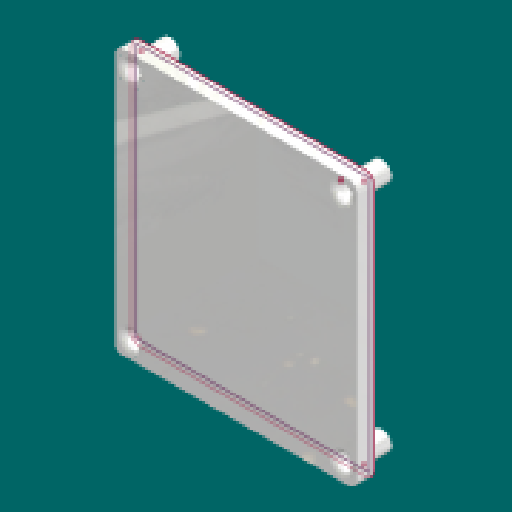
# Autodesk Inventor part: Part_uno_bawah
Saved by Autodesk Inventor 2025.2 (Build 292293000, 293)
## iProperties
Created: 2025-05-06
Part Number: Part_uno_bawah
Material: PPS Plastic
Document SubType Name: Modeling
Designer: ia088
Density: 1.637 g/cm^3
Appearance: Smooth - White
Author: ia088
Autodesk Inventor part; units mm, degrees
ref_plane "YZ Plane" through (0, 0, 0) normal (1, 0, 0) x (0, 1, 0)
ref_plane "XZ Plane" through (0, 0, 0) normal (0, 1, 0) x (-1, 0, 0)
ref_plane "XY Plane" through (0, 0, 0) normal (0, 0, 1) x (1, 0, 0)
ref_plane "Work Plane1" through (0, 0, 0) normal (0, 0, 1) x (1, 0, 0)
sketch "Sketch1" plane through (0, 0, 0) normal (0, 0, 1) x (1, 0, 0)
  line L0 (0, 0) -> (0, -66.04) projected
  line L1 (-53.34, 0) -> (0, 0) projected
  line L2 (-53.34, -66.04) -> (-53.34, 0) projected
  line L3 (-40.386, -66.04) -> (-53.34, -66.04) projected
  line L4 (-37.846, -68.58) -> (-40.386, -66.04) projected
  line L5 (-5.08, -68.58) -> (-37.846, -68.58) projected
  line L6 (-2.54, -66.04) -> (-5.08, -68.58) projected
  line L7 (0, -66.04) -> (-2.54, -66.04) projected
  circle A0 centre (-2.54, -33.02) radius 0.4 projected
  circle A1 centre (-2.54, -35.56) radius 0.4 projected
  circle A2 centre (-2.54, -38.1) radius 0.4 projected
  circle A3 centre (-2.54, -40.64) radius 0.4 projected
  circle A4 centre (-2.54, -43.18) radius 0.4 projected
  circle A5 centre (-2.54, -45.72) radius 0.4 projected
  circle A6 centre (-2.54, -50.8) radius 0.4 projected
  circle A7 centre (-2.54, -53.34) radius 0.4 projected
  circle A8 centre (-2.54, -55.88) radius 0.4 projected
  circle A9 centre (-2.54, -58.42) radius 0.4 projected
  circle A10 centre (-2.54, -60.96) radius 0.4 projected
  circle A11 centre (-2.54, -63.5) radius 0.4 projected
  circle A12 centre (-50.8, -23.876) radius 0.4 projected
  circle A13 centre (-50.8, -26.416) radius 0.4 projected
  circle A14 centre (-50.8, -28.956) radius 0.4 projected
  circle A15 centre (-50.8, -31.496) radius 0.4 projected
  circle A16 centre (-50.8, -34.036) radius 0.4 projected
  circle A17 centre (-50.8, -36.576) radius 0.4 projected
  circle A18 centre (-50.8, -39.116) radius 0.4 projected
  circle A19 centre (-50.8, -41.656) radius 0.4 projected
  circle A20 centre (-50.8, -50.8) radius 0.4 projected
  circle A21 centre (-50.8, -53.34) radius 0.4 projected
  circle A22 centre (-50.8, -55.88) radius 0.4 projected
  circle A23 centre (-50.8, -58.42) radius 0.4 projected
  circle A24 centre (-50.8, -60.96) radius 0.4 projected
  circle A25 centre (-50.8, -63.5) radius 0.4 projected
  circle A26 centre (-12.573, -62.865) radius 0.4 projected
  circle A27 centre (-20.193, -62.865) radius 0.4 projected
  circle A28 centre (-12.573, -60.325) radius 0.4 projected
  circle A29 centre (-20.193, -60.325) radius 0.4 projected
  circle A30 centre (-12.573, -57.785) radius 0.4 projected
  circle A31 centre (-20.193, -57.785) radius 0.4 projected
  circle A32 centre (-12.573, -55.245) radius 0.4 projected
  circle A33 centre (-20.193, -55.245) radius 0.4 projected
  circle A34 centre (-12.573, -52.705) radius 0.4 projected
  circle A35 centre (-20.193, -52.705) radius 0.4 projected
  circle A36 centre (-12.573, -50.165) radius 0.4 projected
  circle A37 centre (-20.193, -50.165) radius 0.4 projected
  circle A38 centre (-12.573, -47.625) radius 0.4 projected
  circle A39 centre (-20.193, -47.625) radius 0.4 projected
  circle A40 centre (-12.573, -45.085) radius 0.4 projected
  circle A41 centre (-20.193, -45.085) radius 0.4 projected
  circle A42 centre (-12.573, -42.545) radius 0.4 projected
  circle A43 centre (-20.193, -42.545) radius 0.4 projected
  circle A44 centre (-12.573, -40.005) radius 0.4 projected
  circle A45 centre (-20.193, -40.005) radius 0.4 projected
  circle A46 centre (-12.573, -37.465) radius 0.4 projected
  circle A47 centre (-20.193, -37.465) radius 0.4 projected
  circle A48 centre (-12.573, -34.925) radius 0.4 projected
  circle A49 centre (-20.193, -34.925) radius 0.4 projected
  circle A50 centre (-12.573, -32.385) radius 0.4 projected
  circle A51 centre (-20.193, -32.385) radius 0.4 projected
  circle A52 centre (-12.573, -29.845) radius 0.4 projected
  circle A53 centre (-20.193, -29.845) radius 0.4 projected
  circle A54 centre (-26.162, -16.383) radius 0.5 projected
  circle A55 centre (-26.162, -21.463) radius 0.5 projected
  circle A56 centre (-39.878, -18.288) radius 0.4 projected
  circle A57 centre (-39.878, -20.828) radius 0.4 projected
  circle A58 centre (-42.418, -20.828) radius 0.4 projected
  circle A59 centre (-42.418, -18.288) radius 0.4 projected
  circle A60 centre (-44.958, -15.748) radius 0.4 projected
  circle A61 centre (-44.958, -18.288) radius 0.4 projected
  circle A62 centre (-44.958, -20.828) radius 0.4 projected
  circle A63 centre (-47.498, -20.828) radius 0.4 projected
  circle A64 centre (-47.498, -18.288) radius 0.4 projected
  circle A65 centre (-47.498, -15.748) radius 0.4 projected
  circle A66 centre (-30.43, -63.64) radius 0.4 projected
  circle A67 centre (-27.89, -63.64) radius 0.4 projected
  circle A68 centre (-25.35, -63.64) radius 0.4 projected
  circle A69 centre (-25.35, -66.18) radius 0.4 projected
  circle A70 centre (-27.89, -66.18) radius 0.4 projected
  circle A71 centre (-30.43, -66.18) radius 0.4 projected
  circle A72 centre (-50.8, -48.26) radius 0.4 projected
  circle A73 centre (-50.8, -21.336) radius 0.4 projected
  circle A74 centre (-50.8, -45.72) radius 0.4 projected
  circle A75 centre (-2.54, -30.48) radius 0.4 projected
  circle A76 centre (-50.8, -18.796) radius 0.4 projected
  circle A77 centre (-2.54, -27.94) radius 0.4 projected
  circle A78 centre (-50.8, -15.24) radius 1.5875 projected
  circle A79 centre (-2.54, -13.97) radius 1.5875 projected
  circle A80 centre (-35.56, -66.04) radius 1.5875 projected
  circle A81 centre (-7.62, -66.04) radius 1.5875 projected
  line L8 (-43.58, 6.35) -> (-32.46, 6.35) projected
  line L9 (-44.04, 6.35) -> (-43.58, 6.35) projected
  line L10 (-32, 6.35) -> (-32.46, 6.35) projected
  line L11 (-32, 5.94) -> (-32, 6.35) projected
  line L12 (-32, 3.85) -> (-32, 5.94) projected
  line L13 (-32, 3.75) -> (-32, -2.65) projected
  line L14 (-32, 5.89) -> (-32, 3.75) projected
  line L15 (-44.04, -2.65) -> (-44.04, 3.75) projected
  line L16 (-44.04, 3.75) -> (-44.04, 5.89) projected
  line L17 (-44.04, 6.35) -> (-44.04, 5.94) projected
  line L18 (-44.04, 5.94) -> (-44.04, 3.85) projected
  line L19 (-53.34, 6.35) -> (-58.34, 6.35)
  line L20 (-58.34, 6.35) -> (31.66, 6.35)
  line L21 (31.66, 6.35) -> (31.66, -73.65)
  line L22 (31.66, -73.65) -> (-58.34, -73.65)
  line L23 (-58.34, -73.65) -> (-58.34, 6.35)
  dimension "d0" = 5
  dimension "d2" = 90
  dimension "d3" = 80
  constraints: 10 end point, 2 horizontal, 2 parallel, 1 perpendicular
  measures "d0" distance of L19.start L19.end
  measures "d2" distance of L21.end L22.end
  measures "d3" distance of L20.end L21.end
ref_plane "Work Plane2" through (0, 0, 0) normal (0, 0, 1) x (1, 0, 0)
sketch "Sketch2" plane through (0, 0, 0) normal (0, 0, 1) x (1, 0, 0)
  point P0 (0, 0)
extrude "Extrusion1" add sketch "Sketch1" along normal blind 5 contours L1 L13 L14 L12 L11 L20 L21 L22 L23 L19 L17 L18 L16 L15 L2 L3 L4 L5 L6 L7 L0 | L0 L7 L6 L5 L4 L3 L2 L1 | L1 L15 L16 L18 L17 L9 L8 L10 L11 L12 L14 L13 | A0 | A1 | A2 | A3 | A4 | A5 | A6 | A7 | A8 | A9 | A10 | A11 | A12 | A13 | A14 | A15 | A16 | A17 | A18 | A19 | A20 | A21 | A22 | A23 | A24 | A25 | A26 | A27 | A28 | A29 | A30 | A31 | A32 | A33 | A34 | A35 | A36 | A37 | A38 | A39 | A40 | A41 | A42 | A43 | A44 | A45 | A46 | A47 | A48 | A49 | A50 | A51 | A52 | A53 | A54 | A55 | A56 | A57 | A58 | A59 | A60 | A61 | A62 | A63 | A64 | A65 | A66 | A67 | A68 | A69 | A70 | A71 | A72 | A73 | A74 | A75 | A76 | A77 | A78 | A79 | A80 | A81
sketch "Sketch3" plane through (0, 0, 0) normal (0, 0, -1) x (-1, 0, 0)
  circle A0 centre (2.54, -13.97) radius 1.5875 projected
  circle A1 centre (50.8, -15.24) radius 1.5875 projected
  circle A2 centre (35.56, -66.04) radius 1.5875 projected
  circle A3 centre (7.62, -66.04) radius 1.5875 projected
  line L0 (53.34, 0) -> (0, 0) construction
  line L1 (0, 0) -> (0, -66.04) construction
  line L2 (0, -66.04) -> (2.54, -66.04) construction
  line L3 (2.54, -66.04) -> (5.08, -68.58) construction
  line L4 (5.08, -68.58) -> (37.846, -68.58) construction
  line L5 (37.846, -68.58) -> (40.386, -66.04) construction
  line L6 (40.386, -66.04) -> (53.34, -66.04) construction
  line L7 (53.34, -66.04) -> (53.34, 0) construction
  line L8 (-0.3, 0.3) -> (53.64, 0.3)
  line L9 (53.64, 0.3) -> (53.64, -66.34)
  line L10 (53.64, -66.34) -> (40.5103, -66.34)
  line L11 (40.5103, -66.34) -> (37.9703, -68.88)
  line L12 (37.9703, -68.88) -> (4.9557, -68.88)
  line L13 (4.9557, -68.88) -> (2.4157, -66.34)
  line L14 (2.4157, -66.34) -> (-0.3, -66.34)
  line L15 (-0.3, -66.34) -> (-0.3, 0.3)
  circle A4 centre (2.54, -13.97) radius 1.2875
  circle A5 centre (50.8, -15.24) radius 1.2875
  circle A6 centre (7.62, -66.04) radius 1.2875
  circle A7 centre (35.56, -66.04) radius 1.2875
  dimension "d6" = 0.3
  dimension "d9" = 0.3
  dimension "d10" = 0.3
  dimension "d11" = 0.3
  dimension "d12" = 0.3
  constraints: 16 end point, 4 centre point, 7 other
  measures "d6" distance between parallel lines of L0 L8
  measures "d9" radial gap between concentric circles of A0 A4
  measures "d10" radial gap between concentric circles of A1 A5
  measures "d11" radial gap between concentric circles of A3 A6
  measures "d12" radial gap between concentric circles of A2 A7
extrude "Extrusion2" cut sketch "Sketch3" against normal blind 3 contours A0 | A1 | A2 | A3 | L8 L9 L10 L11 L12 L13 L14 L15
sketch "Sketch4" plane through (0, 0, 0) normal (0, 0, -1) x (-1, 0, 0)
  circle A0 centre (7.62, -66.04) radius 1.2875 projected
  circle A1 centre (2.54, -13.97) radius 1.2875 projected
  circle A2 centre (50.8, -15.24) radius 1.2875 projected
  circle A3 centre (35.56, -66.04) radius 1.2875 projected
  point P0 (0, 0)
extrude "Extrusion3" add sketch "Sketch4" along normal blind 3
fillet "Fillet1" radius 1 4 edges at (-6.3325, -66.04, 3) (-34.2725, -66.04, 3) (-1.2525, -13.97, 3) (-49.5125, -15.24, 3)
sketch "Sketch5" plane through (0, 0, 0) normal (0, 0, -1) x (-1, 0, 0)
  line L0 (4.9557, -68.88) -> (2.4157, -66.34) projected
  line L1 (2.4157, -66.34) -> (-0.3, -66.34) projected
  line L2 (-0.3, -66.34) -> (-0.3, 0.3) projected
  line L3 (-0.3, 0.3) -> (53.64, 0.3) projected
  line L4 (53.64, 0.3) -> (53.64, -66.34) projected
  line L5 (53.64, -66.34) -> (40.5103, -66.34) projected
  line L6 (40.5103, -66.34) -> (37.9703, -68.88) projected
  line L7 (37.9703, -68.88) -> (4.9557, -68.88) projected
  line L8 (-31.66, 6.35) -> (58.34, 6.35) projected
  line L9 (-31.66, -73.65) -> (-31.66, 6.35) projected
  line L10 (58.34, -73.65) -> (-31.66, -73.65) projected
  line L11 (58.34, 6.35) -> (58.34, -73.65) projected
  line L12 (56.84, 4.85) -> (-30.16, 4.85)
  line L13 (-30.16, 4.85) -> (-30.16, -72.15)
  line L14 (-30.16, -72.15) -> (56.84, -72.15)
  line L15 (56.84, -72.15) -> (56.84, 4.85)
  line L16 (55.14, 1.8) -> (-1.8, 1.8)
  line L17 (-1.8, 1.8) -> (-1.8, -67.84)
  line L18 (-1.8, -67.84) -> (1.7944, -67.84)
  line L19 (1.7944, -67.84) -> (4.3344, -70.38)
  line L20 (4.3344, -70.38) -> (38.5916, -70.38)
  line L21 (38.5916, -70.38) -> (41.1316, -67.84)
  line L22 (41.1316, -67.84) -> (55.14, -67.84)
  line L23 (55.14, -67.84) -> (55.14, 1.8)
  point P0 (0, 0)
  dimension "d16" = 1.5
  dimension "d17" = 1.5
  constraints: 24 end point, 10 other
  measures "d16" distance between parallel lines of L8 L12
  measures "d17" distance between parallel lines of L3 L16
extrude "Extrusion4" cut sketch "Sketch5" against normal blind 3 contours L15 L14 L13 L12
sketch "Sketch6" plane through (-58.34, -73.65, 0) normal (-1, 0, 0) x (0, 0, 1)
  line L0 (0, 80) -> (0, 0) projected
  line L1 (0, 0) -> (5, 0) projected
  line L2 (5, 80) -> (5, 0) projected
  line L3 (0, 80) -> (5, 80) projected
  point P0 (0, 73.65)
extrude "Extrusion5" add sketch "Sketch6" along normal blind 5
sketch "Sketch7" plane through (0, 0, 0) normal (0, 0, -1) x (-1, 0, 0)
  line L0 (63.34, 6.35) -> (63.34, -73.65) projected
  line L1 (56.84, 4.85) -> (56.84, -72.15) projected
  line L2 (56.84, -72.15) -> (61.84, -72.15)
  line L3 (61.84, -72.15) -> (61.84, 4.85)
  line L4 (61.84, 4.85) -> (56.84, 4.85)
  point P0 (0, 0)
  dimension "d23" = 5
  constraints: 6 end point, 2 perpendicular, 1 parallel
  measures "d23" distance of L1.end L2.end
extrude "Extrusion6" cut sketch "Sketch7" against normal up to surface (3 mm away)
sketch "Sketch8" plane through (0, 0, 3) normal (0, 0, -1) x (-1, 0, 0)
  line L0 (-30.16, -72.15) -> (-30.16, 4.85) projected
  line L1 (61.84, -72.15) -> (-30.16, -72.15) projected
  line L2 (61.84, 4.85) -> (-30.16, 4.85) projected
  line L3 (55.14, -67.84) -> (55.14, 1.8) projected
  line L4 (61.84, -72.15) -> (55.84, -72.15)
  line L5 (61.84, -66.15) -> (61.84, -72.15)
  line L6 (61.84, -72.15) -> (55.14, -72.15)
  line L7 (55.14, -72.15) -> (55.14, -65.45)
  line L8 (55.14, -65.45) -> (61.84, -65.45)
  line L9 (61.84, -65.45) -> (61.84, -72.15)
  circle A0 centre (58.49, -68.8) radius 3
  circle A1 centre (58.49, -68.8) radius 1.6
  line L10 (61.84, -72.15) -> (15.84, -72.15)
  line L11 (15.84, -72.15) -> (15.84, 4.85)
  line L12 (-30.16, -72.15) -> (61.84, -72.15)
  circle A2 centre (-26.81, -68.8) radius 3
  line L13 (15.84, -33.65) -> (-30.16, -33.65)
  circle A3 centre (58.49, 1.5) radius 3
  circle A4 centre (58.49, 1.5) radius 1.6
  circle A5 centre (-26.81, 1.5) radius 3
  circle A6 centre (-26.81, -68.8) radius 1.6
  circle A7 centre (-26.81, 1.5) radius 1.6
  point P0 (0, 0)
  dimension "d30" = 6.7
  dimension "d31" = 6
  dimension "d32" = 3.2
  dimension "d33" = 46
  dimension "d34" = 3.2
  dimension "d35" = 3.2
  constraints: 20 end point, 8 centre point, 6 symmetric about line, 4 coincident, 4 midpoint, 2 horizontal, 2 parallel, 1 perpendicular, 1 point on line, 4 other
  measures "d30" distance of L6.end L7.end
  measures "d31" diameter of A0
  measures "d32" diameter of A1
  measures "d33" distance of L1.start L10.end
  measures "d34" diameter of A6
  measures "d35" diameter of A7
extrude "Extrusion7" add sketch "Sketch8" along normal blind 10 contours A0 | A1 | A2 | A3 | A4 | A5 | A6 | A7
sketch "Sketch9" plane through (-58.49, -68.8, -7) normal (0, 0, -1) x (-1, 0, 0)
  circle A0 centre (0, 0) radius 3 projected
  circle A1 centre (0, 0) radius 2
  circle A2 centre (0, 70.3) radius 3 projected
  circle A3 centre (-85.3, 70.3) radius 3 projected
  circle A4 centre (-85.3, 0) radius 3 projected
  circle A5 centre (0, 70.3) radius 2
  circle A6 centre (-85.3, 70.3) radius 2
  circle A7 centre (-85.3, 0) radius 2
  point P0 (-58.49, 68.8)
  dimension "d38" = 1
  dimension "d39" = 1
  dimension "d40" = 1
  dimension "d41" = 1
  constraints: 4 centre point
  measures "d38" radial gap between concentric circles of A0 A1
  measures "d39" radial gap between concentric circles of A2 A5
  measures "d40" radial gap between concentric circles of A3 A6
  measures "d41" radial gap between concentric circles of A4 A7
extrude "Extrusion8" cut sketch "Sketch9" against normal up to surface (12 mm away) contours A1 | A5 | A6 | A7
fillet "Fillet3" radius 2 4 edges at (-56.49, 1.5, 5) (-56.49, -68.8, 5) (28.81, -68.8, 5) (28.81, 1.5, 5)
fillet "Fillet4" radius 1 3 edges at (-55.49, 1.5, 3) (29.81, 1.5, 3) (29.81, -68.8, 3)
sketch "Sketch10" plane through (26.81, -68.8, -7) normal (0, 0, -1) x (-1, 0, 0)
  line L0 (25.01, 70.6) -> (25.01, 0.96) projected
  line L1 (25.01, 0.96) -> (16.81, 0.96)
  line L2 (16.81, 0.96) -> (16.81, -4.85)
  line L3 (-4.85, -4.85) -> (90.15, -4.85) projected
  line L4 (88.65, -3.35) -> (-3.35, -3.35) projected
  line L5 (-3.35, -3.35) -> (-3.35, 73.65) projected
  line L6 (-3.35, 73.65) -> (88.65, 73.65) projected
  line L7 (88.65, 73.65) -> (88.65, -3.35) projected
  line L8 (-4.85, 75.15) -> (90.15, 75.15) projected
  line L9 (-4.85, -4.85) -> (-4.85, 75.15) projected
  line L10 (-4.85, -4.85) -> (90.15, -4.85) projected
  line L11 (90.15, 75.15) -> (90.15, -4.85) projected
  line L12 (16.81, 0.96) -> (16.81, 75.15)
  point P0 (26.81, 68.8)
  dimension "d46" = 8.2
  constraints: 6 end point, 2 perpendicular, 2 point on line, 1 horizontal
  measures "d46" distance of L0.end L1.end
extrude "Extrusion9" cut sketch "Sketch10" against normal up to surface (12 mm away) contours L2 L4 L5 L6 L12 | L2 L3 L9 L8 L12 L6 L5 L4
sketch "Sketch11" plane through (0, 0, 3) normal (0, 0, -1) x (-1, 0, 0)
  line L0 (-10, 4.85) -> (-10, -72.15) projected
  line L1 (61.84, -72.15) -> (-10, -72.15) projected
  line L2 (56.3043, 4.85) -> (-10, 4.85) projected
  line L3 (-10, 6.35) -> (-10, 4.85) projected
  line L4 (-10, 4.85) -> (61.84, 4.85) projected
  line L5 (61.84, 4.85) -> (61.84, -72.15) projected
  line L6 (61.84, -72.15) -> (-10, -72.15) projected
  line L7 (-10, -72.15) -> (-10, -73.65) projected
  line L8 (-10, -73.65) -> (63.34, -73.65) projected
  line L9 (63.34, 6.35) -> (63.34, -73.65) projected
  line L10 (-10, 6.35) -> (63.34, 6.35) projected
  line L11 (-10, -73.65) -> (-8.5, -73.65)
  line L12 (-8.5, -73.65) -> (-8.5, 6.35)
  point P0 (0, 0)
  point P1 (-8.5, -72.15)
  point P2 (-8.5, 4.85)
  dimension "d49" = 1.5
  constraints: 4 end point, 2 point on line, 1 perpendicular
  measures "d49" distance of L7.end L11.end
extrude "Extrusion10" add sketch "Sketch11" along normal up to surface (3 mm away) contours L2 L12 L1 L0
sketch "Sketch12" plane through (0, 0, 3) normal (0, 0, -1) x (-1, 0, 0)
  line L0 (61.84, -72.15) -> (-8.5, -72.15) projected
  circle A0 centre (58.49, -68.8) radius 3 projected
  circle A1 centre (58.49, -68.8) radius 3 projected
  circle A2 centre (58.49, -68.8) radius 2 projected
  circle A3 centre (58.49, -68.8) radius 3 projected
  circle A4 centre (58.49, 1.5) radius 2 projected
  circle A5 centre (58.49, 1.5) radius 3 projected
  circle A6 centre (58.49, -68.8) radius 3
  circle A7 centre (58.49, -68.8) radius 2
  circle A8 centre (58.49, 1.5) radius 3
  circle A9 centre (58.49, 1.5) radius 2
  line L1 (61.84, -72.15) -> (26.67, -72.15)
  line L2 (26.67, -72.15) -> (26.67, 6.35)
  line L3 (-10, 6.35) -> (63.34, 6.35) projected
  circle A10 centre (-5.15, -68.8) radius 3
  circle A11 centre (-5.15, -68.8) radius 2
  circle A12 centre (-5.15, 1.5) radius 3
  circle A13 centre (-5.15, 1.5) radius 2
  point P0 (0, 0)
  dimension "d52" = 35.17
  constraints: 8 centre point, 4 coincident, 4 concentric, 4 end point, 4 symmetric about line, 2 midpoint, 4 other
  measures "d52" distance of L0.start L1.end
extrude "Extrusion11" add sketch "Sketch12" along normal up to surface (10 mm away) contours A10 | A12
sketch "Sketch13" plane through (5.15, -68.8, 3) normal (0, 0, -1) x (-1, 0, 0)
  circle A0 centre (0, 0) radius 2 projected
  circle A1 centre (0, 70.3) radius 2 projected
  point P0 (5.15, 68.8)
extrude "Extrusion12" cut sketch "Sketch13" against normal up to surface (2 mm away)
fillet "Fillet5" radius 2 2 edges at (7.15, 1.5, 5) (7.15, -68.8, 5)
fillet "Fillet6" radius 1 3 edges at (8.15, -68.8, 3) (8.15, 1.5, 3) (-55.49, -68.8, 3)
sketch "Sketch14" plane through (0, 0, 0) normal (0, 0, -1) x (-1, 0, 0)
  line L0 (-10, 6.35) -> (-10, -73.65) projected
  line L1 (-10, -73.65) -> (63.34, -73.65) projected
  line L2 (63.34, 6.35) -> (63.34, -73.65) projected
  line L3 (-10, 6.35) -> (63.34, 6.35) projected
  line L4 (-8.5, 4.85) -> (61.84, 4.85) projected
  line L5 (61.84, 4.85) -> (61.84, -72.15) projected
  line L6 (61.84, -72.15) -> (-8.5, -72.15) projected
  line L7 (-8.5, -72.15) -> (-8.5, 4.85) projected
  line L8 (-10, 6.35) -> (-10, -73.65) projected
  line L9 (-10, -73.65) -> (63.34, -73.65) projected
  line L10 (63.34, 6.35) -> (63.34, -73.65) projected
  line L11 (-10, 6.35) -> (63.34, 6.35) projected
  line L12 (61.34, -73.65) -> (-7, -73.65)
  line L13 (-10, -70.65) -> (-10, 3.35)
  line L14 (-7, 6.35) -> (60.34, 6.35)
  line L15 (63.34, 3.35) -> (63.34, -71.65)
  arc A0 (61.34, -73.65) -> (63.34, -71.65) centre (61.34, -71.65) ccw
  arc A1 (63.34, 3.35) -> (60.34, 6.35) centre (60.34, 3.35) ccw
  arc A2 (-10, -70.65) -> (-7, -73.65) centre (-7, -70.65) ccw
  arc A3 (-7, 6.35) -> (-10, 3.35) centre (-7, 3.35) ccw
  line L16 (-5.5, -72.15) -> (58.84, -72.15)
  line L17 (61.84, -69.15) -> (61.84, 1.85)
  line L18 (58.84, 4.85) -> (-5.5, 4.85)
  line L19 (-8.5, 1.85) -> (-8.5, -69.15)
  arc A4 (61.84, 1.85) -> (58.84, 4.85) centre (58.84, 1.85) ccw
  arc A5 (58.84, -72.15) -> (61.84, -69.15) centre (58.84, -69.15) ccw
  arc A6 (-8.5, -69.15) -> (-5.5, -72.15) centre (-5.5, -69.15) ccw
  arc A7 (-5.5, 4.85) -> (-8.5, 1.85) centre (-5.5, 1.85) ccw
  point P0 (0, 0)
  dimension "d59" = 2
  dimension "d60" = 3
  dimension "d61" = 3
  constraints: 16 end point, 16 point on circle, 16 tangent, 8 centre point, 8 point on line, 5 equal radius, 4 parallel, 2 horizontal, 2 perpendicular
  measures "d59" radius of A0
  measures "d60" radius of A1
  measures "d61" radius of A4
extrude "Extrusion13" cut sketch "Sketch14" against normal blind 5 contours L3 A3 L0 | A2 L1 L0 | L3 L2 A1 | A0 L2 L1
sketch "Sketch15" plane through (0, 0, 0) normal (0, 0, -1) x (-1, 0, 0)
  line L0 (-8.5, 4.85) -> (61.84, 4.85) projected
  line L1 (61.84, 4.85) -> (61.84, -72.15) projected
  line L2 (61.84, -72.15) -> (-8.5, -72.15) projected
  line L3 (-8.5, -72.15) -> (-8.5, 4.85) projected
  line L4 (-5.5, -72.15) -> (58.84, -72.15)
  line L5 (61.84, -69.15) -> (61.84, 1.85)
  line L6 (58.84, 4.85) -> (-5.5, 4.85)
  line L7 (-8.5, 1.85) -> (-8.5, -69.15)
  arc A0 (58.84, -72.15) -> (61.84, -69.15) centre (58.84, -69.15) ccw
  arc A1 (-8.5, -69.15) -> (-5.5, -72.15) centre (-5.5, -69.15) ccw
  arc A2 (61.84, 1.85) -> (58.84, 4.85) centre (58.84, 1.85) ccw
  arc A3 (-5.5, 4.85) -> (-8.5, 1.85) centre (-5.5, 1.85) ccw
  point P0 (0, 0)
  point P1 (58.84, -72.15)
  dimension "d64" = 3
  constraints: 8 end point, 8 point on circle, 8 tangent, 4 centre point, 4 point on line, 3 equal radius, 2 parallel, 1 horizontal, 1 perpendicular
  measures "d64" radius of A0
extrude "Extrusion14" add sketch "Sketch15" against normal up to surface (5 mm away) contours L0 A3 L3 | L0 L1 A2 | A1 L2 L3 | L1 L2 A0
body "Solid1"
